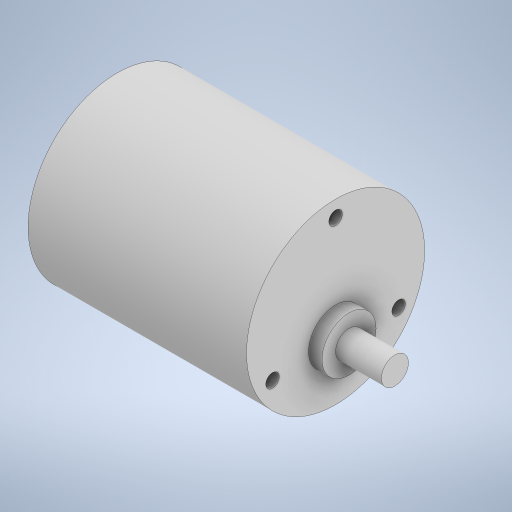
# Autodesk Inventor part: Motor
Saved by Autodesk Inventor 2023 (Build 270158030, 158C)
## iProperties
Created: 2022-06-16
Part Number: Motor
Material: Generic
Document SubType Name: Modeling
Designer: Mlees
Density: 1 g/cm^3
Appearance: Default
Author: Mlees
Autodesk Inventor part; units mm, degrees
ref_plane "YZ Plane" through (0, 0, 0) normal (1, 0, 0) x (0, 1, 0)
ref_plane "XZ Plane" through (0, 0, 0) normal (0, 1, 0) x (-1, 0, 0)
ref_plane "XY Plane" through (0, 0, 0) normal (0, 0, 1) x (1, 0, 0)
sketch "Sketch1" plane through (0, 0, 0) normal (1, 0, 0) x (0, 1, 0)
  circle A0 centre (0, 0) radius 16.5
  dimension "d0" = 33
  constraints: 1 centre point, 1 coincident
  measures "d0" diameter of A0
extrude "Extrusion1" add sketch "Sketch1" along normal blind 40.5
sketch "Sketch2" plane through (40.5, 0, 0) normal (1, 0, 0) x (0, 0, -1)
  circle A0 centre (0, 0) radius 16.5 projected
  circle A1 centre (0, -5.5) radius 5
  constraints: 1 centre point
extrude "Extrusion2" add sketch "Sketch2" along normal blind 2.5 contours A1
sketch "Sketch3" plane through (43, -5.5, 0) normal (1, 0, 0) x (0, 0, -1)
  circle A0 centre (0, 0) radius 2.5
  point P0 (0, 5.5)
  dimension "d7" = 5
  constraints: 1 centre point
  measures "d7" diameter of A0
extrude "Extrusion3" add sketch "Sketch3" along normal blind 8.5
sketch "Sketch4" plane through (40.5, 0, 0) normal (1, 0, 0) x (0, 0, -1)
  circle A0 centre (0, 0) radius 16.5 projected
  circle A1 centre (0, 13.5) radius 1.25
  circle A2 centre (-11.6913, -6.75) radius 1.25
  circle A3 centre (11.6913, -6.75) radius 1.25
  dimension "d11" = 2.5
  dimension "d14" = 360
  constraints: 3 centre point, 7 other
  measures "d11" diameter of A1
extrude "Extrusion4" cut sketch "Sketch4" against normal blind 8.5 contours A1 | A2 | A3
body "Solid1"
